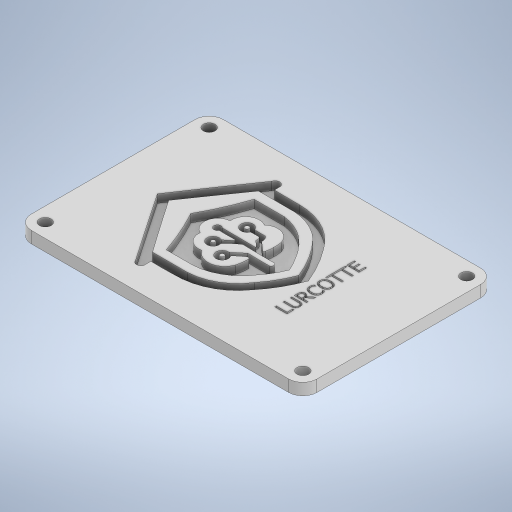
# Autodesk Inventor part: Cover Lurcotte
Saved by Autodesk Inventor 2024 (Build 280153000, 153)
## iProperties
Created: 2025-05-13
Part Number: Cover Lurcotte
Material: Generic
Document SubType Name: Modeling
Designer: chaaa
Density: 1 g/cm^3
Appearance: Default
Author: chaaa
Autodesk Inventor part; units mm, degrees
ref_plane "YZ Plane" through (0, 0, 0) normal (1, 0, 0) x (0, 1, 0)
ref_plane "XZ Plane" through (0, 0, 0) normal (0, 1, 0) x (-1, 0, 0)
ref_plane "XY Plane" through (0, 0, 0) normal (0, 0, 1) x (1, 0, 0)
sketch "Sketch1" plane through (0, 0, 0) normal (0, 1, 0) x (-1, 0, 0)
  arc A0 (-56.6627, 40.3565) -> (-62.6627, 34.3565) centre (-56.6627, 34.3565) ccw
  line L0 (-56.6627, -41.6435) -> (53.3373, -41.6435)
  line L1 (-56.6627, 40.3565) -> (53.3373, 40.3565)
  line L2 (53.3373, -41.6435) -> (-56.6627, -41.6435)
  line L3 (-56.6627, -29.6435) -> (-56.6627, 28.3565)
  line L4 (-62.6627, 34.3565) -> (-62.6627, -35.6435)
  line L5 (59.3373, -35.6435) -> (59.3373, 34.3565)
  line L6 (-50.6627, -35.6435) -> (47.3373, -35.6435)
  line L7 (59.3373, -35.6435) -> (59.3373, 34.3565)
  line L8 (-62.6627, 34.3565) -> (-62.6627, -35.6435)
  circle A1 centre (-56.6627, 34.3565) radius 6
  circle A2 centre (53.3373, 34.3565) radius 1.5
  circle A3 centre (53.3373, 34.3565) radius 6
  circle A4 centre (53.3373, -35.6435) radius 1.5
  circle A5 centre (53.3373, -35.6435) radius 6
  circle A6 centre (-56.6627, -35.6435) radius 1.5
  circle A7 centre (-56.6627, -35.6435) radius 6
  line L9 (53.3373, 28.3565) -> (53.3373, -29.6435)
  line L10 (47.3373, 34.3565) -> (-50.6627, 34.3565)
  circle A8 centre (-56.6627, 34.3565) radius 1.5
  circle A9 centre (-56.6627, 34.3565) radius 1.5
  point P0 (0, 0)
  point P1 (-48.7892, -25.0642)
  point P2 (53.3373, -41.6435)
  constraints: 22 end point, 12 point on circle, 10 centre point, 5 coincident, 4 parallel, 2 horizontal, 2 perpendicular, 1 tangent
extrude "Extrusion1" add sketch "Sketch1" along normal blind 5
sketch "Sketch2" plane through (0, 5, 0) normal (0, 1, 0) x (1, 0, 0)
  circle A0 centre (-53.3373, -34.3565) radius 1.5 projected
  circle A1 centre (-53.3373, -34.3565) radius 2.5
  circle A2 centre (-53.3373, 35.6435) radius 1.5 projected
  circle A3 centre (-53.3373, 35.6435) radius 2.5
  circle A4 centre (56.6627, 35.6435) radius 1.5 projected
  circle A5 centre (56.6627, 35.6435) radius 2.5
  circle A6 centre (56.6627, -34.3565) radius 2.5
  point P0 (0, 0)
  dimension "d2" = 5
  dimension "d3" = 5
  dimension "d4" = 5
  dimension "d5" = 5
  constraints: 4 centre point, 3 coincident
  measures "d2" diameter of A1
  measures "d3" diameter of A3
  measures "d4" diameter of A5
  measures "d5" diameter of A6
extrude "Extrusion2" cut sketch "Sketch2" against normal blind 3.5 contours A0 | A1 | A3 | A5 | A6
sketch "Sketch3" plane through (0, 5, 0) normal (0, 1, 0) x (1, 0, 0)
  arc A0 (2.325, -4.2217) -> (-1.2471, -7.2304) centre (14.3642, -22.1401) ccw
  arc A1 (-2.9502, -6.217) -> (1.3987, -2.5578) centre (-216.8996, 252.469) ccw
  arc A2 (3.3378, -16.0517) -> (11.4807, -8.5153) centre (-7.4204, 3.7396) ccw
  arc A3 (3.0421, -9.7059) -> (3.7264, -4.412) centre (-12.8467, -4.961) ccw
  arc A4 (3.7264, -4.412) -> (2.325, -4.2217) centre (2.9454, -4.9082) ccw
  arc A5 (1.3987, -2.5578) -> (10.8484, -2.6554) centre (9.9014, 363.3812) ccw
  arc A6 (-2.9238, -0.3774) -> (10.8484, -0.5466) centre (8.3647, 357.9854) ccw
  circle A7 centre (-3.3371, -8.8052) radius 0.9007
  arc A8 (-2.9502, -6.217) -> (-1.2471, -7.2304) centre (-3.3371, -8.8052) ccw
  arc A9 (-2.9238, -0.3774) -> (-7.9356, -4.719) centre (13.849, -24.8031) ccw
  arc A10 (-6.1638, -0.7271) -> (-6.4311, -0.2498) centre (-6.546, -0.6276) ccw
  arc A11 (11.4807, -8.5153) -> (16.4487, 0.0903) centre (-12.6612, 11.1587) ccw
  arc A12 (15.8557, -15.22) -> (15.8557, -15.22) centre (-1.1432, 0.0903) ccw
  arc A13 (13.6096, -12.0692) -> (20.4903, 0.0903) centre (-22.1276, 16.1798) ccw
  arc A14 (15.8557, -15.22) -> (24.5731, 0.0903) centre (-24.0349, 17.6299) ccw
  arc A15 (0.7536, 1.2405) -> (0.7536, 1.6759) centre (0.6929, 1.4582) ccw
  arc A16 (3.949, 1.2738) -> (0.0432, 4.6511) centre (-35.2622, -40.1264) ccw
  arc A17 (0.0432, 4.6511) -> (-1.1432, 7.5361) centre (-3.2272, 4.9926) ccw
  arc A18 (-1.6316, 3.7854) -> (-2.1999, 5.859) centre (-3.6223, 4.3545) ccw
  arc A19 (-2.1999, 5.859) -> (-5.8334, 5.859) centre (-4.0167, -53.7238) ccw
  arc A20 (-5.7916, 7.5941) -> (-1.1432, 7.5361) centre (-2.738, 66.0511) ccw
  arc A21 (4.5345, 8.5466) -> (-5.5262, 11.4184) centre (-1.4035, 6.8029) ccw
  arc A22 (5.881, 14.5561) -> (-4.3995, 18.7333) centre (-7.1344, -2.7369) ccw
  arc A23 (10.0999, 16.5176) -> (-4.3995, 22.7345) centre (-5.5262, 0.0903) ccw
  arc A24 (5.881, 14.5561) -> (5.881, 14.5561) centre (-5.5262, 0.0903) ccw
  arc A25 (4.7644, 5.2073) -> (4.5345, 8.5466) centre (-14.2838, 5.5737) ccw
  arc A26 (4.4121, 1.9092) -> (4.7644, 5.2073) centre (-11.0455, 5.2279) ccw
  arc A27 (16.4487, 0.0903) -> (14.0101, 4.7956) centre (-12.2113, -11.779) ccw
  arc A28 (14.0101, 4.7956) -> (5.881, 14.5561) centre (-14.1065, -10.3558) ccw
  arc A29 (-9.5211, -11.3681) -> (3.0421, -9.7059) centre (-3.6476, -7.453) ccw
  arc A30 (-4.3995, 22.7345) -> (-4.7587, 22.68) centre (-1.1432, 0.0903) ccw
  circle A31 centre (-8.2981, 6.7864) radius 0.9274
  arc A32 (-5.7916, 7.5941) -> (-5.8334, 5.859) centre (-8.2981, 6.7864) ccw
  arc A33 (0.7536, 1.2405) -> (-13.3845, 1.3647) centre (-318.0204, -35455.8006) ccw
  arc A34 (-5.5262, 11.4184) -> (-14.3613, 5.6224) centre (-8.5217, 6.3527) ccw
  circle A35 centre (-10.4487, -5.5549) radius 0.8359
  arc A36 (-9.1487, -3.2474) -> (-7.9356, -4.719) centre (-10.4487, -5.5549) ccw
  arc A37 (-6.1638, -0.7271) -> (-9.1487, -3.2474) centre (582.5104, -700.9511) ccw
  arc A38 (-13.1525, -0.2498) -> (-6.4311, -0.2498) centre (-9.7918, 85.9094) ccw
  arc A39 (-13.3845, 1.3647) -> (-13.1525, -0.2498) centre (-14.558, 0.3722) ccw
  arc A40 (-14.3613, 5.6224) -> (-16.4114, -5.1725) centre (-14.0212, -0.0343) ccw
  arc A41 (-3.0899, -26.0947) -> (15.8557, -15.22) centre (-5.5262, 0.0903) ccw
  arc A42 (-6.1638, -18.7516) -> (3.3378, -16.0517) centre (-6.8209, 1.6299) ccw
  arc A43 (-4.3995, -22.554) -> (13.6096, -12.0692) centre (-5.5262, 0.0903) ccw
  arc A44 (-16.9329, -18.7516) -> (-16.3222, -18.7502) centre (-16.9329, 116.166) ccw
  line L0 (-16.3222, -18.7516) -> (-6.1638, -18.7516)
  line L1 (-17.2717, -18.7516) -> (-6.1638, -18.7516)
  line L2 (-4.3995, -22.554) -> (-19.3393, -22.5343)
  arc A45 (-19.8876, -29.3081) -> (-16.3222, -29.3081) centre (-18.1049, -28.6961) ccw
  line L3 (-16.3222, -29.3081) -> (-16.3222, -26.2923)
  arc A46 (-16.3222, -26.2923) -> (-3.0899, -26.0947) centre (-11.8655, 118.4344) ccw
  arc A47 (-16.4114, -5.1725) -> (-9.5211, -11.3681) centre (-10.7478, -5.8031) ccw
  line L4 (-17.2714, 18.7333) -> (-4.3995, 18.7333)
  line L5 (-4.7587, 22.68) -> (-19.3392, 22.6992)
  arc A48 (-16.3222, 26.4878) -> (-5.6121, 26.3882) centre (-6.3763, 520.4893) ccw
  line L6 (-16.3222, 29.1605) -> (-16.3222, 26.4878)
  arc A49 (-16.3222, 29.1605) -> (-20.126, 29.1605) centre (-18.2241, 28.6639) ccw
  arc A50 (-19.3392, 22.6992) -> (-34.5275, 0.8552) centre (1845.5191, -1290.1572) ccw
  arc A51 (-20.126, 29.1605) -> (-39.9001, 0.0903) centre (1549.832, -1060.0097) ccw
  arc A52 (-19.3392, 22.6992) -> (-35.0526, 0.0903) centre (1845.5191, -1290.1572) ccw
  arc A53 (-25.4811, -0.0434) -> (-17.2714, 18.7333) centre (-119.3488, 52.1813) ccw
  arc A54 (-17.2717, -18.7516) -> (-25.4811, -0.0434) centre (-132.8267, -58.3034) ccw
  arc A55 (-35.0526, 0.0903) -> (-19.3393, -22.5343) centre (1135.7625, 796.48) ccw
  arc A56 (-39.9001, 0.0903) -> (-19.8876, -29.3081) centre (2870.2125, 1959.5929) ccw
  arc A57 (10.8484, -2.6554) -> (10.8484, -0.5466) centre (10.3399, -1.601) ccw
  arc A58 (24.5731, 0.0903) -> (15.8557, 15.4006) centre (-36.4882, -24.5401) ccw
  arc A59 (15.8557, 15.4006) -> (-5.6121, 26.3882) centre (-5.5262, 0.0903) ccw
  arc A60 (20.4903, 0.0903) -> (10.0999, 16.5176) centre (-27.5607, -18.8026) ccw
  arc A61 (3.949, 1.2738) -> (4.4121, 1.9092) centre (3.8331, 1.8448) ccw
  arc A62 (0.7536, 1.6759) -> (-1.6316, 3.7854) centre (-18.4135, -17.5931) ccw
  line L7 (26.8233, -17.2049) -> (26.8233, 17.6016) construction
  line L8 (26.8233, 17.6016) -> (32.3061, 17.6016) construction
  line L9 (32.3061, 17.6016) -> (32.3061, -17.2049) construction
  line L10 (32.3061, -17.2049) -> (26.8233, -17.2049) construction
  line L11 (32.1952, -13.6236) -> (32.1952, -16.672)
  line L12 (32.1952, -16.672) -> (26.9342, -16.672)
  line L13 (26.9342, -16.672) -> (26.9342, -15.9728)
  line L14 (26.9342, -15.9728) -> (31.5727, -15.9728)
  line L15 (31.5727, -15.9728) -> (31.5727, -13.6236)
  line L16 (31.5727, -13.6236) -> (32.1952, -13.6236)
  spline S0 degree 2 poles (32.3061, -11.2361) (32.3061, -11.7008) (32.063, -12.3915) (31.82, -12.6345) knots 0 0 0 1 2 2 2
  spline S1 degree 2 poles (31.82, -12.6345) (31.5472, -12.9116) (30.7798, -13.1376) (30.217, -13.1376) knots 0 0 0 1 2 2 2
  line L17 (30.217, -13.1376) -> (26.9342, -13.1376)
  line L18 (26.9342, -13.1376) -> (26.9342, -12.4384)
  line L19 (26.9342, -12.4384) -> (30.217, -12.4384)
  spline S2 degree 2 poles (30.217, -12.4384) (30.5836, -12.4384) (31.0782, -12.3446) (31.2786, -12.2124) knots 0 0 0 1 2 2 2
  spline S3 degree 2 poles (31.2786, -12.2124) (31.4917, -12.0717) (31.7092, -11.5857) (31.7092, -11.2361) knots 0 0 0 1 2 2 2
  spline S4 degree 2 poles (31.7092, -11.2361) (31.7092, -10.9078) (31.4917, -10.3962) (31.2786, -10.2555) knots 0 0 0 1 2 2 2
  spline S5 degree 2 poles (31.2786, -10.2555) (31.0782, -10.1234) (30.5879, -10.0296) (30.234, -10.0296) knots 0 0 0 1 2 2 2
  line L20 (30.234, -10.0296) -> (26.9342, -10.0296)
  line L21 (26.9342, -10.0296) -> (26.9342, -9.3304)
  line L22 (26.9342, -9.3304) -> (30.217, -9.3304)
  spline S6 degree 2 poles (30.217, -9.3304) (30.767, -9.3304) (31.5514, -9.5521) (31.82, -9.8334) knots 0 0 0 1 2 2 2
  spline S7 degree 2 poles (31.82, -9.8334) (32.0673, -10.085) (32.3061, -10.7501) (32.3061, -11.2361) knots 0 0 0 1 2 2 2
  line L23 (32.1952, -4.2569) -> (32.1952, -5.165)
  line L24 (32.1952, -5.165) -> (30.1019, -6.8277)
  line L25 (30.1019, -6.8277) -> (30.1019, -7.6293)
  line L26 (30.1019, -7.6293) -> (32.1952, -7.6293)
  line L27 (32.1952, -7.6293) -> (32.1952, -8.3285)
  line L28 (32.1952, -8.3285) -> (26.9342, -8.3285)
  line L29 (26.9342, -8.3285) -> (26.9342, -6.9727)
  spline S8 degree 2 poles (26.9342, -6.9727) (26.9342, -6.5208) (27.0322, -5.9111) (27.2113, -5.634) knots 0 0 0 1 2 2 2
  spline S9 degree 2 poles (27.2113, -5.634) (27.3903, -5.3569) (27.9488, -5.0371) (28.3624, -5.0371) knots 0 0 0 1 2 2 2
  spline S10 degree 2 poles (28.3624, -5.0371) (28.938, -5.0371) (29.7182, -5.6255) (29.9058, -6.1285) knots 0 0 0 1 2 2 2
  line L30 (29.9058, -6.1285) -> (32.1952, -4.2569)
  spline S11 degree 2 poles (28.4178, -5.7661) (28.1876, -5.7661) (27.8337, -5.9282) (27.7186, -6.0987) knots 0 0 0 1 2 2 2
  spline S12 degree 2 poles (27.7186, -6.0987) (27.6206, -6.2479) (27.5396, -6.6444) (27.5396, -6.9343) knots 0 0 0 1 2 2 2
  line L31 (27.5396, -6.9343) -> (27.5396, -7.6293)
  line L32 (27.5396, -7.6293) -> (29.5178, -7.6293)
  line L33 (29.5178, -7.6293) -> (29.5178, -7.0153)
  spline S13 degree 2 poles (29.5178, -7.0153) (29.5178, -6.7126) (29.4112, -6.2309) (29.2449, -6.0646) knots 0 0 0 1 2 2 2
  spline S14 degree 2 poles (29.2449, -6.0646) (29.1, -5.9111) (28.6907, -5.7661) (28.4178, -5.7661) knots 0 0 0 1 2 2 2
  spline S15 degree 2 poles (32.289, -1.7841) (32.289, -2.2957) (31.9437, -3.1612) (31.5983, -3.4767) knots 0 0 0 1 2 2 2
  spline S16 degree 2 poles (31.5983, -3.4767) (31.2573, -3.7922) (30.234, -4.1375) (29.5689, -4.1375) knots 0 0 0 1 2 2 2
  spline S17 degree 2 poles (29.5689, -4.1375) (28.9081, -4.1375) (27.9275, -3.8007) (27.5651, -3.481) knots 0 0 0 1 2 2 2
  spline S18 degree 2 poles (27.5651, -3.481) (27.2113, -3.1655) (26.8404, -2.3043) (26.8404, -1.7713) knots 0 0 0 1 2 2 2
  spline S19 degree 2 poles (26.8404, -1.7713) (26.8404, -1.507) (26.9171, -1.0423) (26.9768, -0.8462) knots 0 0 0 1 2 2 2
  spline S20 degree 2 poles (26.9768, -0.8462) (27.0322, -0.6756) (27.19, -0.3218) (27.2838, -0.147) knots 0 0 0 1 2 2 2
  line L34 (27.2838, -0.147) -> (28.1279, -0.147)
  line L35 (28.1279, -0.147) -> (28.1279, -0.2024)
  spline S21 degree 2 poles (28.1279, -0.2024) (28.0426, -0.2962) (27.8039, -0.5861) (27.6888, -0.795) knots 0 0 0 1 2 2 2
  spline S22 degree 2 poles (27.6888, -0.795) (27.5779, -0.9954) (27.4372, -1.4686) (27.4372, -1.7756) knots 0 0 0 1 2 2 2
  spline S23 degree 2 poles (27.4372, -1.7756) (27.4372, -2.1124) (27.7144, -2.7135) (27.9787, -2.9395) knots 0 0 0 1 2 2 2
  spline S24 degree 2 poles (27.9787, -2.9395) (28.2473, -3.1612) (29.0616, -3.4085) (29.5689, -3.4085) knots 0 0 0 1 2 2 2
  spline S25 degree 2 poles (29.5689, -3.4085) (30.1104, -3.4085) (30.8906, -3.1484) (31.1592, -2.9225) knots 0 0 0 1 2 2 2
  spline S26 degree 2 poles (31.1592, -2.9225) (31.4193, -2.7008) (31.6836, -2.1081) (31.6836, -1.7756) knots 0 0 0 1 2 2 2
  spline S27 degree 2 poles (31.6836, -1.7756) (31.6836, -1.4729) (31.5344, -0.957) (31.4235, -0.7566) knots 0 0 0 1 2 2 2
  spline S28 degree 2 poles (31.4235, -0.7566) (31.3127, -0.5648) (31.0825, -0.2791) (31.0015, -0.1981) knots 0 0 0 1 2 2 2
  line L36 (31.0015, -0.1981) -> (31.0015, -0.147)
  line L37 (31.0015, -0.147) -> (31.8371, -0.147)
  spline S29 degree 2 poles (31.8371, -0.147) (31.9181, -0.3218) (32.0673, -0.6287) (32.1355, -0.8462) knots 0 0 0 1 2 2 2
  spline S30 degree 2 poles (32.1355, -0.8462) (32.2123, -1.0764) (32.289, -1.4686) (32.289, -1.7841) knots 0 0 0 1 2 2 2
  spline S31 degree 2 poles (27.5353, 4.2273) (27.8849, 4.5257) (28.9081, 4.8583) (29.5647, 4.8583) knots 0 0 0 1 2 2 2
  spline S32 degree 2 poles (29.5647, 4.8583) (30.2042, 4.8583) (31.2402, 4.5343) (31.5898, 4.2273) knots 0 0 0 1 2 2 2
  spline S33 degree 2 poles (31.5898, 4.2273) (31.9565, 3.9033) (32.3061, 3.0463) (32.3061, 2.5305) knots 0 0 0 1 2 2 2
  spline S34 degree 2 poles (32.3061, 2.5305) (32.3061, 1.9975) (31.9437, 1.1448) (31.5898, 0.8336) knots 0 0 0 1 2 2 2
  spline S35 degree 2 poles (31.5898, 0.8336) (31.2402, 0.5309) (30.2127, 0.2069) (29.5647, 0.2069) knots 0 0 0 1 2 2 2
  spline S36 degree 2 poles (29.5647, 0.2069) (28.9039, 0.2069) (27.8977, 0.5352) (27.5353, 0.8379) knots 0 0 0 1 2 2 2
  spline S37 degree 2 poles (27.5353, 0.8379) (27.1857, 1.1448) (26.8233, 2.0018) (26.8233, 2.5305) knots 0 0 0 1 2 2 2
  spline S38 degree 2 poles (26.8233, 2.5305) (26.8233, 3.0676) (27.1985, 3.9289) (27.5353, 4.2273) knots 0 0 0 1 2 2 2
  spline S39 degree 2 poles (29.5647, 4.1292) (29.0445, 4.1292) (28.2388, 3.9033) (27.9744, 3.6986) knots 0 0 0 1 2 2 2
  spline S40 degree 2 poles (27.9744, 3.6986) (27.7016, 3.4897) (27.4287, 2.9014) (27.4287, 2.5347) knots 0 0 0 1 2 2 2
  spline S41 degree 2 poles (27.4287, 2.5347) (27.4287, 2.1553) (27.693, 1.584) (27.9744, 1.3665) knots 0 0 0 1 2 2 2
  spline S42 degree 2 poles (27.9744, 1.3665) (28.243, 1.1576) (29.0531, 0.9359) (29.5647, 0.9359) knots 0 0 0 1 2 2 2
  spline S43 degree 2 poles (29.5647, 0.9359) (30.6007, 0.9359) (31.7007, 1.8057) (31.7007, 2.5347) knots 0 0 0 1 2 2 2
  spline S44 degree 2 poles (31.7007, 2.5347) (31.7007, 3.2638) (30.6007, 4.1292) (29.5647, 4.1292) knots 0 0 0 1 2 2 2
  line L38 (32.1952, 6.8536) -> (27.5566, 6.8536)
  line L39 (27.5566, 6.8536) -> (27.5566, 5.0885)
  line L40 (27.5566, 5.0885) -> (26.9342, 5.0885)
  line L41 (26.9342, 5.0885) -> (26.9342, 9.3178)
  line L42 (26.9342, 9.3178) -> (27.5566, 9.3178)
  line L43 (27.5566, 9.3178) -> (27.5566, 7.5528)
  line L44 (27.5566, 7.5528) -> (32.1952, 7.5528)
  line L45 (32.1952, 7.5528) -> (32.1952, 6.8536)
  line L46 (32.1952, 11.0786) -> (27.5566, 11.0786)
  line L47 (27.5566, 11.0786) -> (27.5566, 9.3135)
  line L48 (27.5566, 9.3135) -> (26.9342, 9.3135)
  line L49 (26.9342, 9.3135) -> (26.9342, 13.5429)
  line L50 (26.9342, 13.5429) -> (27.5566, 13.5429)
  line L51 (27.5566, 13.5429) -> (27.5566, 11.7778)
  line L52 (27.5566, 11.7778) -> (32.1952, 11.7778)
  line L53 (32.1952, 11.7778) -> (32.1952, 11.0786)
  line L54 (32.1952, 14.0758) -> (26.9342, 14.0758)
  line L55 (26.9342, 14.0758) -> (26.9342, 17.3671)
  line L56 (26.9342, 17.3671) -> (27.5566, 17.3671)
  line L57 (27.5566, 17.3671) -> (27.5566, 14.775)
  line L58 (27.5566, 14.775) -> (28.9976, 14.775)
  line L59 (28.9976, 14.775) -> (28.9976, 17.1923)
  line L60 (28.9976, 17.1923) -> (29.6201, 17.1923)
  line L61 (29.6201, 17.1923) -> (29.6201, 14.775)
  line L62 (29.6201, 14.775) -> (31.5727, 14.775)
  line L63 (31.5727, 14.775) -> (31.5727, 17.3671)
  line L64 (31.5727, 17.3671) -> (32.1952, 17.3671)
  line L65 (32.1952, 17.3671) -> (32.1952, 14.0758)
  point P0 (0, 0)
  point P1 (0.3556, 3.3859)
  point P2 (-13.0268, 2.206)
  point P3 (11.8944, 28.4757)
  point P4 (16.4487, 0.0903)
  point P5 (-34.5275, 0.8552)
  constraints: 129 point on circle, 63 centre point, 14 end point, 4 coincident, 2 point on line, 1 collinear, 1 concentric, 1 parallel, 1 tangent, 2 other
extrude "Extrusion3" cut sketch "Sketch3" against normal blind 3.5 contours A42 A24 A54 A53 A22 A28 A27 A11 A2 | A42 L0 A12 A54 A24 | A54 A12 A53 A24 | A12 L0 A44 L1 A54 | A54 A53 A12 | A43 A13 A60 A23 A12 A58 A14 | A12 A41 A46 L3 A45 A56 A51 A49 L6 A48 A59 L5 A50 A52 A55 L2 | A53 A12 L4 A22 A24 | A53 L4 A12 | A12 A58 A14 | L11 L12 L13 L14 L15 L16 | S0 S1 L17 L18 L19 S2 S3 S4 S5 L20 L21 L22 S6 S7 | L23 L24 L25 L26 L27 L28 L29 S8 S9 S10 L30 | S15 S16 S17 S18 S19 S20 L34 L35 S21 S22 S23 S24 S25 S26 S27 S28 L36 L37 S29 S30 | S31 S32 S33 S34 S35 S36 S37 S38 | L38 L39 L40 L41 L48 L43 L44 L45 | L48 L41 L42 L43 | L42 L49 L50 L51 L52 L53 L46 L47 | L54 L55 L56 L57 L58 L59 L60 L61 L62 L63 L64 L65
body "Solid1"
